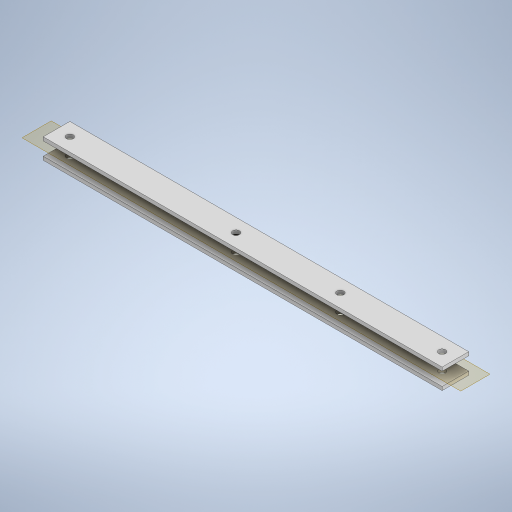
# Autodesk Inventor part: ArmPart1
Saved by Autodesk Inventor 2024 (Build 280153000, 153)
## iProperties
Created: 2024-01-04
Part Number: ArmPart1
Material: Generic
Document SubType Name: Modeling
Designer: student
Density: 1 g/cm^3
Appearance: Default
Author: student
Autodesk Inventor part; units mm, degrees
ref_plane "YZ Plane" through (0, 0, 0) normal (1, 0, 0) x (0, 1, 0)
ref_plane "XZ Plane" through (0, 0, 0) normal (0, 1, 0) x (-1, 0, 0)
ref_plane "XY Plane" through (0, 0, 0) normal (0, 0, 1) x (1, 0, 0)
sketch "Sketch1" plane through (0, 0, 0) normal (0, 1, 0) x (-1, 0, 0)
  line L0 (0, 0) -> (381, 0)
  line L1 (381, 0) -> (381, -25.4)
  line L2 (381, -25.4) -> (0, -25.4)
  line L3 (0, -25.4) -> (0, 0)
  dimension "d0" = 381
  dimension "d1" = 25.4
  constraints: 8 end point, 2 parallel, 1 horizontal, 1 perpendicular
  measures "d0" distance of L1.end L2.end
  measures "d1" distance of L0.end L1.end
extrude "Extrusion1" add sketch "Sketch1" along normal blind 3.429
sketch "Sketch2" plane through (0, 3.429, 0) normal (0, 1, 0) x (1, 0, 0)
  line L0 (0, 25.4) -> (-381, 25.4) projected
  line L1 (-50.8, 25.4) -> (-89.0524, 25.4)
  line L2 (-89.0524, 25.4) -> (-89.0524, 21.7932)
  line L3 (-89.0524, 21.7932) -> (-50.8, 21.7932)
  line L4 (-50.8, 21.7932) -> (-50.8, 25.4)
  line L5 (0, 0) -> (0, 25.4) projected
  line L6 (-127.1524, 25.4) -> (-257.6322, 25.4)
  line L7 (-257.6322, 25.4) -> (-257.6322, 21.7932)
  line L8 (-257.6322, 21.7932) -> (-127.1524, 21.7932)
  line L9 (-127.1524, 21.7932) -> (-127.1524, 25.4)
  point P0 (-89.0524, 23.5966)
  dimension "d4" = 38.2524
  dimension "d5" = 3.6068
  dimension "d6" = 50.8
  dimension "d7" = 38.1
  dimension "d8" = 3.6068
  dimension "d9" = 130.4798
  constraints: 16 end point, 4 parallel, 2 horizontal, 2 perpendicular, 2 point on line, 1 midpoint
  measures "d4" distance of L3.end L2.end
  measures "d5" distance of L2.end L1.end
  measures "d6" distance between parallel lines of L5 L4
  measures "d7" distance from line of point (-89.052, 23.597) L9
  measures "d8" distance of L6.end L7.end
  measures "d9" distance of L7.end L8.end
extrude "Extrusion2" add sketch "Sketch2" along normal blind 12.5984
sketch "Sketch3" plane through (0, 16.0274, 0) normal (0, 1, 0) x (1, 0, 0)
  line L0 (-381, 25.4) -> (-381, 0) projected
  line L1 (-257.6322, 25.4) -> (-381, 25.4) projected
  line L2 (-381, 0) -> (0, 0) projected
  line L3 (0, 0) -> (0, 25.4) projected
  line L4 (0, 25.4) -> (-381, 25.4)
  line L5 (-381, 25.4) -> (-381, 0)
  line L6 (-381, 0) -> (0, 0)
  line L7 (0, 0) -> (0, 25.4)
  constraints: 8 end point, 2 parallel, 1 horizontal, 1 perpendicular
extrude "Extrusion3" add sketch "Sketch3" along normal blind 3.429
sketch "Sketch5" plane through (0, 19.4564, 0) normal (0, 1, 0) x (1, 0, 0)
  line L0 (0, 0) -> (0, 25.4) projected
  line L1 (0, 25.4) -> (-381, 25.4) projected
  point P0 (-12.7, 12.7)
  point P1 (-245.745, 25.4)
  dimension "d18" = 12.7
  dimension "d19" = 12.7
  measures "d18" distance from line of L0 point (-12.7, 12.7)
  measures "d19" distance from line of L1 point (-12.7, 12.7)
hole "Hole1" at (-12.7, 19.4564, -12.7) direction (0, -1, 0) diameter 6.5024 end through all
sketch "Sketch6" plane through (0, 19.4564, 0) normal (0, 1, 0) x (1, 0, 0)
  line L0 (0, 25.4) -> (-381, 25.4) projected
  line L1 (-381, 25.4) -> (-381, 0) projected
  point P0 (-209.55, 12.7)
  point P1 (-245.745, 25.4)
  dimension "d36" = 12.7
  dimension "d37" = 171.45
  measures "d36" distance from line of L0 point (-209.55, 12.7)
  measures "d37" distance from line of L1 point (-209.55, 12.7)
hole "Hole2" at (-209.55, 19.4564, -12.7) direction (0, -1, 0) diameter 6.5024 end through all
sketch "Sketch7" plane through (0, 19.4564, 0) normal (0, 1, 0) x (1, 0, 0)
  line L0 (0, 25.4) -> (-381, 25.4) projected
  line L1 (-381, 25.4) -> (-381, 0) projected
  point P0 (0, 0)
  point P1 (-368.3, 12.7)
  point P2 (-279.654, 25.4)
  dimension "d38" = 12.7
  dimension "d39" = 12.7
  measures "d38" distance from line of L0 point (-368.3, 12.7)
  measures "d39" distance from line of L1 point (-368.3, 12.7)
hole "Hole3" at (-368.3, 19.4564, -12.7) direction (0, -1, 0) diameter 6.5024 end through all
sketch "Sketch10" plane through (0, 19.4564, 0) normal (0, 1, 0) x (1, 0, 0)
  line L0 (0, 25.4) -> (-381, 25.4) projected
  point P0 (0, 0)
  point P1 (-109.9578, 12.7)
  point P2 (-245.745, 25.4)
  dimension "d64" = 12.7
  measures "d64" distance from line of L0 point (-109.958, 12.7)
hole "Hole6" at (-109.9578, 19.4564, -12.7) direction (0, -1, 0) diameter 6.5024 end through all
ref_plane "Work Plane2" through (0, 9.7282, 0) normal (0, 1, 0) x (1, 0, 0)
sketch "Sketch11" plane through (0, 0, 0) normal (0, -1, 0) x (1, 0, 0)
  line L0 (-279.654, -25.4) -> (-279.654, -13.3858) projected
  line L1 (-279.654, -13.3858) -> (-245.745, -13.3858) projected
  line L2 (-245.745, -25.4) -> (-245.745, -13.3858) projected
  line L3 (-245.745, -13.3858) -> (-279.654, -13.3858)
  line L4 (-279.654, -13.3858) -> (-279.654, -25.4)
  line L5 (-279.654, -25.4) -> (-245.745, -25.4)
  line L6 (-245.745, -25.4) -> (-245.745, -13.3858)
  point P0 (0, 0)
  constraints: 8 end point, 2 parallel, 1 horizontal, 1 perpendicular
extrude "Extrusion5" cut sketch "Sketch11" against normal blind 7.9375
body "Solid1"
